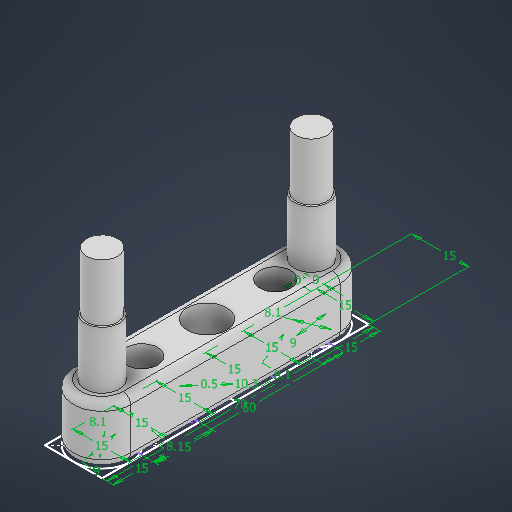
# Autodesk Inventor part: Gear_Holder_2
Saved by Autodesk Inventor 2026.2 (Build 302298000, 298)
## iProperties
Created: 2025-12-19
Part Number: Gear_Holder_2
Material: Generic
Document SubType Name: Modeling
Designer: Cobble
Density: 1 g/cm^3
Appearance: Default
Author: Cobble
Autodesk Inventor part; units mm, degrees
ref_plane "YZ Plane" through (0, 0, 0) normal (1, 0, 0) x (0, 1, 0)
ref_plane "XZ Plane" through (0, 0, 0) normal (0, 1, 0) x (-1, 0, 0)
ref_plane "XY Plane" through (0, 0, 0) normal (0, 0, 1) x (1, 0, 0)
sketch "Sketch1" plane through (0, 0, 0) normal (0, 0, 1) x (1, 0, 0)
  line L0 (0, -70) -> (15, -70)
  line L1 (15, -70) -> (15, 0)
  line L2 (15, 0) -> (0, 0)
  line L3 (0, 0) -> (0, -70)
  line L4 (15, -35) -> (0, -35)
  line L5 (0, -9.5012) -> (15, -9.5012)
  line L6 (15, -9.5012) -> (15, -59.5012)
  line L7 (15, -59.5012) -> (0, -59.5012)
  line L8 (0, -59.5012) -> (0, -9.5012)
  line L9 (0, -9.5012) -> (15, -59.5012) construction
  line L10 (15, -9.5012) -> (0, -59.5012) construction
  line L11 (7.5, -34.5012) -> (7.5349, -35)
  circle A0 centre (7.5349, -35) radius 5.15
  line L12 (0, -70) -> (15, -70)
  line L13 (15, -70) -> (15, -55)
  line L14 (15, -55) -> (0, -55) construction
  line L15 (0, -55) -> (0, -70)
  line L16 (0, 0) -> (15, 0)
  line L17 (15, 0) -> (15, -15)
  line L18 (15, -15) -> (0, -15) construction
  line L19 (0, -15) -> (0, 0)
  line L20 (15, -55) -> (0, -70) construction
  line L21 (0, 0) -> (15, -15) construction
  circle A1 centre (7.5, -62.5) radius 7.5
  circle A2 centre (7.5, -7.5) radius 7.5
  line L22 (0, -59.5012) -> (15, -59.5012)
  line L23 (15, -59.5012) -> (15, -44.5012)
  line L24 (15, -44.5012) -> (0, -44.5012)
  line L25 (0, -44.5012) -> (0, -59.5012)
  line L26 (15, -9.5012) -> (0, -9.5012)
  line L27 (0, -9.5012) -> (0, -24.5012)
  line L28 (0, -24.5012) -> (15, -24.5012)
  line L29 (15, -24.5012) -> (15, -9.5012)
  line L30 (0, -24.5012) -> (15, -9.5012) construction
  line L31 (0, -59.5012) -> (15, -44.5012) construction
  circle A3 centre (7.5, -52.0012) radius 4.05
  circle A4 centre (7.5, -17.0012) radius 4.05
  circle A5 centre (7.5, -62.5) radius 4.05
  circle A6 centre (7.5, -7.5) radius 4.05
  circle A7 centre (7.5, -7.5) radius 4.5
  circle A8 centre (7.5, -62.5) radius 4.5
  point P0 (15, -7.5)
  point P1 (0, -7.5)
  point P2 (0, -62.5)
  point P3 (15, -62.5)
  dimension "d0" = 15
  dimension "d1" = 70
  dimension "d2" = 15
  dimension "d3" = 50
  dimension "d4" = 0.5
  dimension "d5" = 10.3
  dimension "d6" = 15
  dimension "d7" = 15
  dimension "d8" = 15
  dimension "d9" = 15
  dimension "d10" = 15
  dimension "d11" = 15
  dimension "d12" = 15
  dimension "d14" = 8.1
  dimension "d15" = 8.1
  dimension "d16" = 8.1
  dimension "d17" = 8.1
  dimension "d18" = 15
  dimension "d19" = 0
  dimension "d20" = 0
  dimension "d27" = 9
  dimension "d28" = 9
  constraints: 64 end point, 12 parallel, 9 centre point, 7 midpoint, 6 horizontal, 6 perpendicular, 5 coincident, 2 tangent, 1 point on line
  measures "d0" distance of L3.start L1.end
  measures "d1" distance of L1.end L0.end
  measures "d2" distance of L6.end L8.start
  measures "d3" distance of L6.start L6.end
  measures "d4" distance of L11.start L11.end
  measures "d5" diameter of A0
  measures "d6" distance of L14.end L14.start
  measures "d7" distance of L14.start L12.end
  measures "d8" distance of L18.start L18.end
  measures "d9" distance of L16.end L18.start
  measures "d10" distance of L24.end L24.start
  measures "d11" distance of L24.start L23.start
  measures "d12" distance of L28.end L28.start
  measures "d14" diameter of A3
  measures "d15" diameter of A4
  measures "d16" diameter of A5
  measures "d17" diameter of A6
  measures "d18" horizontal distance of L1.end L8.end
  measures "d19" distance of point (0, 0) L3.start
  measures "d20" distance of point (0, 0) L3.start
  measures "d27" diameter of A7
  measures "d28" diameter of A8
extrude "Extrusion1" add sketch "Sketch1" along normal blind 15 contours A1 L7 A8 | L3 L7 A1 | A1 L7 L1 | L3 L24 L1 L7 A1 A3 | A1 A3 L7 A8 | A8 L7 A5 | L7 A5 A8 | A3 A1 | A1 A3 | L3 L4 A0 L1 L24 | L3 L28 L1 L4 A0 | L3 L5 A2 A4 L1 L28 | L3 A2 L5 | L5 A2 L1 | A2 L5 A7 | L5 A7 A2 A4 | A7 L5 A6 | L5 A6 A7 | A4 A2 | A2 A4
extrude "Extrusion2" add sketch "Sketch1" along normal blind 45 contours A5 L7 | L7 A5 | A6 L5 | L5 A6
extrude "Extrusion3" cut sketch "Sketch1" along normal blind 15 contours A3 A1 | A1 A3 | A4 A2 | A2 A4
extrude "Extrusion4" add sketch "Sketch1" along normal blind 30 contours A8 L7 A5 | L7 A5 A8 | A5 L7 | L7 A5 | A7 L5 A6 | L5 A6 A7 | A6 L5 | L5 A6
fillet "Fillet1" radius 2 8 edges at (7.5, 0, 15) (0, -35, 15) (7.5, -70, 15) (15, -35, 15) (7.5, 0, 0) (0, -35, 0) (7.5, -70, 0) (15, -35, 0)
body "Solid1"
